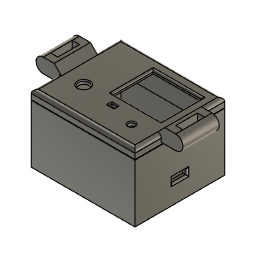
enclosure v12 (Autodesk Fusion 360 design; units mm, degrees)
Autodesk Fusion 360 part; units mm, degrees
sketch "top" plane through (0, 0, 0) normal (0, 0, 1) x (1, 0, 0)
  line L0 (26.35, -22.5) -> (-26.35, -22.5)
  line L1 (-26.35, -22.5) -> (-26.35, 22.5)
  line L2 (-26.35, 22.5) -> (26.35, 22.5)
  line L3 (26.35, 22.5) -> (26.35, -22.5)
  line L4 (26.35, -22.5) -> (-26.35, 22.5) construction
  line L5 (-26.35, -22.5) -> (26.35, 22.5) construction
  line L6 (28.65, -24.8) -> (-28.65, -24.8)
  line L7 (-28.65, -24.8) -> (-28.65, 24.8)
  line L8 (-28.65, 24.8) -> (28.65, 24.8)
  line L9 (28.65, 24.8) -> (28.65, -24.8)
  line L10 (-4.3, 18.2) -> (22.35, 18.2)
  line L11 (22.35, 18.2) -> (22.35, -4.05)
  line L12 (22.35, -4.05) -> (-4.3, -4.05)
  line L13 (-4.3, -4.05) -> (-4.3, 18.2)
  line L14 (0.07, -9.05) -> (3.17, -9.05)
  line L15 (3.17, -9.05) -> (3.17, -10.93)
  line L16 (3.17, -10.93) -> (0.07, -10.93)
  line L17 (0.07, -10.93) -> (0.07, -9.05)
  circle A0 centre (15.8, -13.85) radius 1.65
  circle A1 centre (-16.35, -8.13) radius 3
  line L18 (24.05, -20.2) -> (-24.05, -20.2)
  line L19 (-24.05, -20.2) -> (-24.05, 20.2)
  line L20 (-24.05, 20.2) -> (24.05, 20.2)
  line L21 (24.05, 20.2) -> (24.05, -20.2)
  line L22 (28.65, 9.7223) -> (40.65, 9.7223)
  line L23 (40.65, 9.7223) -> (40.65, -10.2777)
  line L24 (40.65, -10.2777) -> (28.65, -10.2777)
  line L25 (28.65, -10.2777) -> (28.65, 9.7223)
  line L26 (0, 24.8) -> (0, -24.8) construction
  line L27 (-28.65, 9.881) -> (-40.65, 9.881)
  line L28 (-40.65, 9.881) -> (-40.65, -10.119)
  line L29 (-40.65, -10.119) -> (-28.65, -10.119)
  line L30 (-28.65, -10.119) -> (-28.65, 9.881)
  line L31 (36.65, -6.2777) -> (32.65, -6.2777)
  line L32 (32.65, -6.2777) -> (32.65, 5.7223)
  line L33 (32.65, 5.7223) -> (36.65, 5.7223)
  line L34 (36.65, 5.7223) -> (36.65, -6.2777)
  line L35 (-36.65, -6.119) -> (-32.65, -6.119)
  line L36 (-32.65, -6.119) -> (-32.65, 5.881)
  line L37 (-32.65, 5.881) -> (-36.65, 5.881)
  line L38 (-36.65, 5.881) -> (-36.65, -6.119)
  dimension "d1" = 52.7
  dimension "d2" = 45
  dimension "d3" = -2.3
  dimension "d4" = 26.65
  dimension "d5" = 22.25
  dimension "d9" = 4
  dimension "d10" = 3.1
  dimension "d11" = 1.88
  dimension "d12" = 5
  dimension "d13" = 4.37
  dimension "d14" = 3.3
  dimension "d15" = 6
  dimension "d16" = 18.45
  dimension "d19" = 7
  dimension "d20" = 11.37
  dimension "d21" = 8.15
  dimension "d22" = 10.98
  dimension "d60" = 2.3
  dimension "d150" = 12
  dimension "d152" = 20
  dimension "d159" = 14.5223
  dimension "d160" = 14.919
  dimension "d162" = 4
  dimension "d163" = -4
  constraint horizontal L0
  constraint perpendicular L0 L1
  constraint parallel L0 L2
  constraint parallel L1 L3
  constraint coincident L4 origin
  constraint coincident L5 origin
  constraint horizontal L10
  constraint vertical L11
  constraint horizontal L12
  constraint vertical L13
  constraint horizontal L14
  constraint vertical L15
  constraint horizontal L16
  constraint vertical L17
  constraint horizontal L22
  constraint vertical L23
  constraint horizontal L24
  constraint vertical L25
  constraint coincident L9 L22.start
  constraint midpoint L8 L26.start
  constraint midpoint L6 L26.end
  constraint horizontal L27
  constraint vertical L28
  constraint horizontal L29
  constraint vertical L30
  constraint coincident L7 L27.start
  constraint equal L22 L27
  constraint equal L23 L28
  measures "d1" distance of L1.end L2.end
  measures "d2" distance of L0.end L1.end
  measures "d4" distance of L10.start L10.end
  measures "d5" distance of L10.start L12.end
  measures "d9" distance of L3 L11
  measures "d10" distance of L14.start L14.end
  measures "d11" distance of L14.start L16.end
  measures "d12" distance of L12 L14
  measures "d13" distance of L12.end L17
  measures "d14" diameter of A0
  measures "d15" diameter of A1
  measures "d16" distance of L0 L12
  measures "d19" distance of L1 A1
  measures "d20" distance of L0 A1
  measures "d21" distance of L12 A0
  measures "d22" distance of L15 A0
  measures "d150" distance of L22.start L22.end
  measures "d152" distance of L22.end L23.end
  measures "d159" distance of L6 L24
  measures "d160" distance of L8 L27
extrude "Extrude2" add sketch "top" against normal blind 2 contours L0 L1 L2 L3 | L6 L7 L8 L9 L25 L30 | L18 L19 L20 L21 makes body 1
extrude "Extrude3" add sketch "top" against normal blind 5 contours L6 L7 L8 L9 L25 L30 bodies 1
extrude "Extrude8" add sketch "top" against normal blind 13 contours L0 L1 L2 L3 bodies 1
sketch "bottom" plane through (0, 0, -5) normal (0, 0, -1) x (1, 0, 0)
  line L0 (26.35, -22.5) -> (-26.35, -22.5)
  line L1 (-26.35, -22.5) -> (-26.35, 22.5)
  line L2 (-26.35, 22.5) -> (26.35, 22.5)
  line L3 (28.65, 24.8) -> (-28.65, 24.8)
  circle A0 centre (0, 0) radius 5
  line L4 (26.35, -22.5) -> (-26.35, -22.5)
  line L5 (-26.35, -22.5) -> (-26.35, 22.5)
  line L6 (-26.35, 22.5) -> (26.35, 22.5)
  line L7 (26.35, 22.5) -> (26.35, -22.5)
  line L8 (-28.65, -24.8) -> (28.65, -24.8)
  line L9 (28.65, -24.8) -> (28.65, 24.8)
  line L10 (28.65, 24.8) -> (-28.65, 24.8)
  line L11 (-28.65, 24.8) -> (-28.65, -24.8)
  line L12 (0, 0) -> (5, 0) construction
  line L13 (5, 0) -> (7.5, 0) construction
  line L14 (0, -2) -> (7.5, -2)
  arc A1 (7.5, -2) -> (7.5, 2) centre (7.5, 0) ccw
  line L15 (7.5, 2) -> (0, 2)
  arc A2 (0, 2) -> (0, -2) centre (0, 0) ccw
  line L16 (0, 0) -> (7.5, 0) construction
  dimension "d67" = 10
  dimension "d131" = 2.5
  dimension "d132" = 2
  constraint coincident A0.centre L12.start
  constraint horizontal L12
  constraint coincident A0 L12.end
  constraint parallel L12 L13
  constraint tangent L14 A1
  constraint tangent A1 L15
  constraint parallel L14 L15
  constraint tangent L15 A2
  constraint tangent L14 A2
  constraint coincident L13.end A1.centre
  constraint parallel L13 L16
  measures "d67" diameter of A0
  measures "d131" distance of L12.end L13.end
  measures "d132" radius of A1
extrude "Extrude9" add sketch "bottom" along normal blind 32 from surface at 0.25 separate body contours L3 L8 L9 L10 L11 makes body 2
extrude "Extrude10" add sketch "bottom" along normal blind 2.5 from surface at 29.75 contours L0 L1 L2 L4 L5 L6 L7 bodies 2
fillet "Fillet5" radius 1 4 edges at (-4.3, 7.075, 0) (9.025, -4.05, 0) (22.35, 7.075, 0) (9.025, 18.2, 0) on bodies 1
sketch "bottom_backplate" plane through (0, 0, -34.75) normal (0, 0, 1) x (-1, 0, 0)
  line L0 (-4.5826, -2) -> (-7.5, -2)
  arc A0 (-7.5, 2) -> (-7.5, -2) centre (-7.5, 0) ccw
  line L1 (-7.5, 2) -> (-4.5826, 2)
  line L2 (-26.35, 22.5) -> (-26.35, -22.5)
  line L3 (-26.35, -22.5) -> (26.35, -22.5)
  line L4 (26.35, -22.5) -> (26.35, 22.5)
  line L5 (26.35, 22.5) -> (-26.35, 22.5)
  line L6 (26.35, -22.5) -> (-26.35, -22.5)
  line L7 (-26.35, -22.5) -> (-26.35, 22.5)
  line L8 (-26.35, 22.5) -> (26.35, 22.5)
  line L9 (26.35, 22.5) -> (26.35, -22.5)
  line L10 (-4.5826, -2) -> (-4.5826, 2)
  line L11 (-4.5826, -2) -> (-7.5, -2)
  line L12 (-4.5826, 2) -> (-7.5, 2)
  arc A1 (-7.5, 2) -> (-7.5, -2) centre (-7.5, 0) ccw
  dimension "d137" = 2
  constraint horizontal L6
  constraint vertical L7
  constraint horizontal L8
  constraint vertical L9
  constraint coincident L2.start L5.end
  constraint coincident L3.end L4.start
  constraint coincident L0.start L10.start
  constraint coincident L1.end L10.end
  constraint coincident L0.end A0.end
  constraint coincident A0.start L1.start
  measures "d137" radius of A1
extrude "Extrude11" add sketch "bottom_backplate" along normal blind 3 bodies 2
sketch "right" plane through (28.65, 0, 0) normal (1, 0, 0) x (0, 1, 0)
  line L0 (24.8, -5.25) -> (-24.8, -5.25)
  line L1 (-24.8, -5.25) -> (-24.8, -37.25)
  line L2 (-24.8, -37.25) -> (24.8, -37.25)
  line L3 (24.8, -37.25) -> (24.8, -5.25)
  line L4 (3.9119, -24.15) -> (-3.8381, -24.15)
  line L5 (-3.8381, -24.15) -> (-3.8381, -26.95)
  line L6 (-3.8381, -26.95) -> (3.9119, -26.95)
  line L7 (3.9119, -26.95) -> (3.9119, -24.15)
  line L8 (3.9119, -24.15) -> (-3.8381, -26.95) construction
  line L9 (-3.8381, -24.15) -> (3.9119, -26.95) construction
  line L10 (22.5, -5) -> (-22.5, -5)
  line L11 (-22.5, -5) -> (-22.5, -13)
  line L12 (-22.5, -13) -> (22.5, -13)
  line L13 (22.5, -13) -> (22.5, -5)
  line L14 (24.8, 0) -> (-24.8, 0)
  line L15 (-24.8, 0) -> (-24.8, -5)
  line L16 (-24.8, -5) -> (24.8, -5)
  line L17 (24.8, -5) -> (24.8, 0)
  line L18 (-4.05, -1) -> (18.2, -1)
  line L19 (18.2, -1) -> (18.2, -2)
  line L20 (18.2, -2) -> (-4.05, -2)
  line L21 (-4.05, -2) -> (-4.05, -1)
  line L22 (-2, -34.75) -> (2, -34.75)
  line L23 (2, -34.75) -> (2, -31.75)
  line L24 (2, -31.75) -> (-2, -31.75)
  line L25 (-2, -31.75) -> (-2, -34.75)
  point P0 (0.0369, -25.55)
  dimension "d140" = 7.75
  dimension "d141" = 2.8
  dimension "d145" = 24.15
  dimension "d146" = 0.8
  constraint horizontal L4
  constraint perpendicular L4 L5
  constraint parallel L4 L6
  constraint parallel L5 L7
  constraint coincident L8 P0
  constraint coincident L9 P0
  measures "d140" distance of L5.end L6.end
  measures "d141" distance of L4.end L5.end
  measures "d145" distance of L4 L14
extrude "Extrude12" cut sketch "right" against normal blind 3 contours L4 L5 L6 L7 bodies 2
extrude "Extrude13" add sketch "top" along normal blind 4 and the other way blind 4 contours L9 L22 L23 L24 L25 | L7 L27 L28 L29 L30 bodies 1
extrude "Extrude14" add 1 faces at (28.65, 3.0556, 2.6667) along direction (-1, 0, 0) blind 2 on bodies 1 bodies 1
extrude "Extrude15" add 1 faces at (-28.65, -3.4523, 2.6667) along direction (1, 0, 0) blind 2 on bodies 1 bodies 1
fillet "Fillet6" radius 4 4 edges at (40.65, -0.2777, 4) (40.65, -0.2777, -4) (-40.65, -0.119, 4) (-40.65, -0.119, -4) on bodies 1
chamfer "Chamfer1" distance 4 angle 45 2 edges at (26.65, -0.2777, 4) (-26.65, -0.119, 4) on bodies 1
fillet "Fillet7" radius 2 6 edges at (0, -24.8, 0) (-28.65, -17.4595, 0) (-28.65, 17.3405, 0) (0, 24.8, 0) (28.65, 17.2612, 0) (28.65, -17.5388, 0) on bodies 1
fillet "Fillet8" radius 1 4 edges at (28.65, 0.0369, -24.15) (28.65, -3.8381, -25.55) (28.65, 0.0369, -26.95) (28.65, 3.9119, -25.55) on bodies 2
fillet "Fillet9" radius 0.5 1 edges at (-19.147, -7.0452, 0) on bodies 1
fillet "Fillet10" radius 0.5 5 edges at (1.62, -9.05, 0) (14.2617, -13.2533, 0) (0.07, -9.99, 0) (1.62, -10.93, 0) (3.17, -9.99, 0) on bodies 1
named bodies: "top", "bottom"
